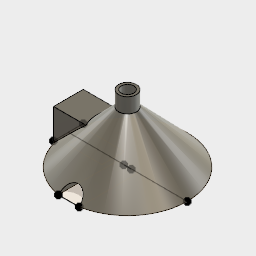
Slip Joint Base v5 (Autodesk Fusion 360 design; units mm, degrees)
Autodesk Fusion 360 part; units mm, degrees
sketch "Sketch1" plane through (0, 0, 0) normal (0, 1, 0) x (1, 0, 0)
  circle A0 centre (0, 0) radius 6
  dimension "d2" = 12
  measures "d2" diameter of A0
extrude "Extrude1" add sketch "Sketch1" along normal blind 3 makes body 1
sketch "Sketch2" plane through (0, 3, 0) normal (0, 1, 0) x (-1, 0, 0)
  circle A0 centre (0, 0) radius 6
  circle A1 centre (0, 0) radius 4.25
  dimension "d5" = 8.5
  measures "d5" diameter of A1
extrude "Extrude2" add sketch "Sketch2" along normal blind 7 bodies 1
ref_plane "WorkPlane1" through (0, -35, 0) normal (0, -1, 0) x (-1, 0, 0)
sketch "Sketch3" plane through (0, -35, 0) normal (0, -1, 0) x (1, 0, 0)
  circle A0 centre (0, 0) radius 40
  dimension "d9" = 80
  measures "d9" diameter of A0
loft "Loft1" add profiles "Sketch3" section 1 section 2 face at (-0.9566, 0, 0.2914) on bodies 1 bodies 1
sketch "Sketch4" plane through (0, 3, 0) normal (0, 1, 0) x (-1, 0, 0)
  circle A0 centre (0, 0) radius 4.25
  circle A1 centre (0, 0) radius 2.5
  dimension "d10" = 5
  measures "d10" diameter of A1
extrude "Extrude7" cut sketch "Sketch4" against normal blind 60 contours A1 bodies 1
extrude "Extrude3" cut sketch "Sketch4" against normal blind 54 contours A1 bodies 1
sketch "Sketch5" plane through (0, 0, 0) normal (0, 0, 1) x (1, 0, 0)
  circle A0 centre (0, -35) radius 7
  line L0 (2.5, -35) -> (-2.5, -35)
extrude "Extrude10" cut sketch "Sketch5" along normal blind 60 bodies 1
extrude "Extrude4" cut sketch "Sketch5" along normal blind 43 bodies 1
sketch "Sketch6" plane through (0, 0, 0) normal (0, 1, 0) x (1, 0, 0)
sketch "Sketch7" plane through (0, 0, 0) normal (0, 0, 1) x (1, 0, 0)
  circle A0 centre (25, 25) radius 3
  dimension "d15" = 6
  measures "d15" diameter of A0
extrude "Extrude5" add sketch "Sketch7" along normal blind 100 separate body makes body 2
move_body "Move1" bodies 2 to x (1, 0, 0) y (0, 1, 0) z (0, 0, 1) at (-25, -50, 0)
move_body "Align1" bodies 2 to x (1, 0, 0) y (0, 0, -1) z (0, 1, 0) at (0, -135, -25)
move_body "Move2" bodies 2 to x (0, 0, -1) y (-1, 0, 0) z (0, 1, 0) at (-138, -132, -6)
sketch "Sketch8" plane through (0, 0, 0) normal (1, 0, 0) x (0, 0, -1)
  line L0 (40, -35) -> (-39.3827, -35)
  line L1 (-39.3827, -35) -> (-39.3827, -15)
  line L2 (-39.3827, -15) -> (40, -15)
  line L3 (40, -15) -> (40, -35)
  line L4 (0.3086, -15) -> (-9.6914, -15)
  line L5 (0.3086, -15) -> (10.3086, -15)
  line L6 (10.3086, -15) -> (10.3086, -35)
  line L7 (-9.6914, -15) -> (-9.6914, -35)
  dimension "d18" = 20
  dimension "d19" = 10
  dimension "d20" = 10
  measures "d18" distance of L0.start L2.end
  measures "d19" distance of L4.start L4.end
  measures "d20" distance of L4.start L5.end
extrude "Extrude6" add sketch "Sketch8" against normal blind 40 contours L0 L2 L4 L5 L6 L7 bodies 1
sketch "Sketch9" plane through (0, -35, 0) normal (0, -1, 0) x (1, 0, 0)
  arc A0 (-7, 39.3827) -> (-38.8082, 9.6914) centre (0, 0) ccw
  line L0 (-38.8082, 9.6914) -> (-40, 9.6914)
  line L1 (-40, 9.6914) -> (-40, -10.3086)
  line L2 (-40, -10.3086) -> (-38.6488, -10.3086)
  arc A1 (0, -2.5) -> (2.5, 0) centre (0, 0) ccw
  line L3 (0, -2.5) -> (0, 9.6914)
  line L4 (0, 9.6914) -> (-7, 9.6914)
  line L5 (-40, -0.3086) -> (-40, 7.1914)
  line L6 (-40, -0.3086) -> (-40, -7.8086)
  line L7 (-40, -10.3086) -> (-33, -10.3086)
  line L8 (-40, 9.6914) -> (-33, 9.6914)
  line L9 (-33, 9.6914) -> (-33, -10.3086)
  line L10 (-40, -7.8086) -> (-10, -7.8086)
  line L11 (-40, 7.1914) -> (-10, 7.1914)
  line L12 (-10, 7.1914) -> (-10, -7.8086)
  circle A2 centre (0, 0) radius 2.5
  line L13 (-7, 9.6914) -> (-7, 39.3827)
  arc A3 (-38.6488, -10.3086) -> (7, 39.3827) centre (0, 0) ccw
  line L14 (7, 39.3827) -> (7, 0)
  line L15 (7, 0) -> (2.5, 0)
  dimension "d25" = 7.5
  dimension "d26" = 7.5
  dimension "d27" = 7
  dimension "d28" = 7
  dimension "d29" = 30
  dimension "d30" = 30
  measures "d25" distance of L5.start L5.end
  measures "d26" distance of L5.start L6.end
  measures "d27" distance of L1.end L7.end
  measures "d28" distance of L0.end L8.end
  measures "d29" distance of L6.end L10.end
  measures "d30" distance of L5.end L11.end
extrude "Extrude9" cut sketch "Sketch9" against normal blind 17.5 contours L9 L10 L11 L12 bodies 1
extrude "Extrude8" cut sketch "Sketch9" against normal blind 48 contours L3 A2 bodies 1
move_body "Align2" bodies 2 to x (1, 0, 0) y (0, 1, 0) z (0, 0, 1) at (63, 107, 5.6914)
move_body "Move3" bodies 2 to x (1, 0, 0) y (0, 1, 0) z (0, 0, 1) at (-90, 0, 0)
combine "Combine1" operation cut target body 1 tool bodies 2 keep tools
sketch "Sketch10" plane through (0, 0, 0) normal (0, 0, 1) x (1, 0, 0)
  line L0 (2.5, -28.4617) -> (2.5, -35)
  line L1 (2.5, -35) -> (7, -35)
  arc A0 (7, -35) -> (2.5, -28.4617) centre (0, -35) ccw
  circle A1 centre (0, -35) radius 7
extrude "Extrude11" cut sketch "Sketch10" along normal blind 32 contours L0 L1 A1 bodies 1
move_face "OffsetFaces1" offset -2 1 faces at (-35.3333, -25.1495, -3.3049) on bodies 1
sketch "Sketch11" plane through (0, 0, 0) normal (0, 0, 1) x (1, 0, 0)
  line L0 (6, 10) -> (-6, 10)
  line L1 (-6, 10) -> (6, 10)
  line L2 (-40, -35) -> (40, -35)
  line L3 (-40, -35) -> (-40, -15)
  line L4 (-7, -35) -> (7, -35)
  line L5 (-2.5, -35) -> (2.5, -35)
  line L6 (0, -35) -> (0, 10)
  point P0 (6, 10)
  point P1 (-40, -35)
  point P2 (-7, -35)
  point P3 (7, -35)
  point P4 (-2.5, -35)
  point P5 (2.5, -35)
  dimension "d40" = 80
  dimension "d41" = 12
  dimension "d42" = 20
  dimension "d43" = 14
  dimension "d44" = 5
  dimension "d45" = 45
  measures "d40" distance of P1 L2.end
  measures "d41" distance of L0.end P0
  measures "d42" distance of P1 L3.end
  measures "d43" distance of P2 P3
  measures "d44" distance of P4 P5
  measures "d45" distance of L6.start L6.end
sketch "Sketch12" plane through (0, -35, 0) normal (0, -1, 0) x (1, 0, 0)
  line L0 (-10, -7.8086) -> (-33, -7.8086)
  line L1 (-33, -7.8086) -> (-33, 7.1914)
  line L2 (-33, 7.1914) -> (-10, 7.1914)
  line L3 (-10, 7.1914) -> (-10, -7.8086)
  line L4 (-2.5, 0) -> (-7, 0)
  line L5 (-7, 0) -> (-7, 39.3827)
  arc A0 (-7, 39.3827) -> (-38.8082, 9.6914) centre (0, 0) ccw
  line L6 (-38.8082, 9.6914) -> (-40, 9.6914)
  line L7 (-40, 9.6914) -> (-40, -10.3086)
  line L8 (-40, -10.3086) -> (-38.6488, -10.3086)
  arc A1 (-38.6488, -10.3086) -> (7, 39.3827) centre (0, 0) ccw
  line L9 (7, 39.3827) -> (7, 0)
  line L10 (7, 0) -> (2.5, 0)
  arc A2 (-2.5, 0) -> (2.5, 0) centre (0, 0) ccw
  line L11 (-7, 39.3827) -> (7, 39.3827)
  line L12 (-2.5, 0) -> (2.5, 0)
  line L13 (-40, -10.3086) -> (-40, 9.6914)
  line L14 (-40, -0.3086) -> (40, 0)
  dimension "d46" = 80
  dimension "d47" = 20
  dimension "d48" = 5
  dimension "d49" = 14
  measures "d46" distance of L14.start L14.end
  measures "d47" distance of L7.end L6.end
  measures "d48" distance of L4.start L10.end
  measures "d49" distance of L5.end A1.end
hidden bodies 2
named bodies: "Slip Joint Base", "M6 Threaded Rod"
